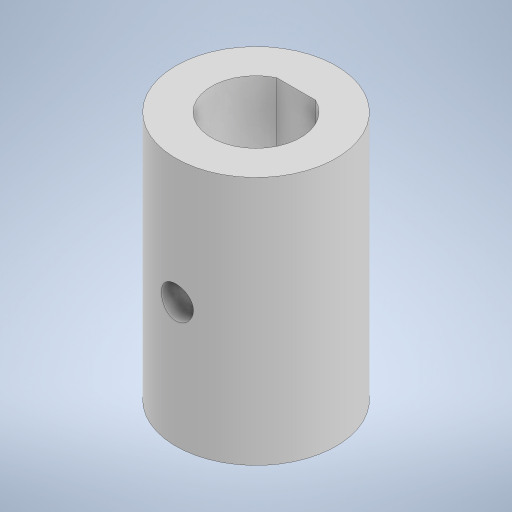
# Autodesk Inventor part: shaft_connector
Saved by Autodesk Inventor 2024.2 (Build 282272000, 272)
## iProperties
Created: 2024-02-07
Part Number: shaft_connector
Material: Generic
Document SubType Name: Modeling
Designer: tamiz
Density: 1 g/cm^3
Appearance: Default
Author: tamiz
Autodesk Inventor part; units mm, degrees
ref_plane "YZ Plane" through (0, 0, 0) normal (1, 0, 0) x (0, 1, 0)
ref_plane "XZ Plane" through (0, 0, 0) normal (0, 1, 0) x (-1, 0, 0)
ref_plane "XY Plane" through (0, 0, 0) normal (0, 0, 1) x (1, 0, 0)
sketch "Sketch1" plane through (0, 0, 0) normal (0, 1, 0) x (-1, 0, 0)
  circle A0 centre (0, 0) radius 5
  circle A1 centre (0, 0) radius 9
  dimension "d0" = 10
  dimension "d1" = 4
  constraints: 2 centre point, 1 coincident
  measures "d0" diameter of A0
  measures "d1" radial gap between concentric circles of A0 A1
extrude "Extrusion1" add sketch "Sketch1" along normal blind 28
sketch "Sketch2" plane through (0, 0, 0) normal (0, 0, 1) x (1, 0, 0)
  line L0 (9, 28) -> (-9, 28) projected
  line L1 (0, 28) -> (0, 0)
  circle A0 centre (0, 14) radius 1.8
  dimension "d4" = 3.6
  constraints: 2 end point, 2 midpoint, 1 centre point, 1 vertical
  measures "d4" diameter of A0
extrude "Extrusion2" cut sketch "Sketch2" along normal mid plane 20
sketch "Sketch4" plane through (0, 28, 0) normal (0, 1, 0) x (1, 0, 0)
  line L0 (2.1794, 4.5) -> (-2.1794, 4.5)
  arc A0 (2.1794, 4.5) -> (-2.1794, 4.5) centre (0, 0) ccw
  constraints: 2 end point, 2 point on circle, 1 centre point
extrude "Extrusion3" add sketch "Sketch4" against normal blind 11
body "Solid1"
